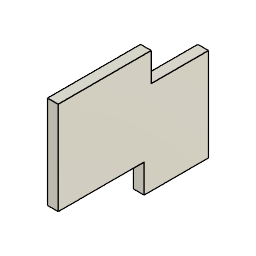
right_side_face_plate (Autodesk Fusion 360 design; units mm, degrees)
part number: 2025-10-03-12-31-24-970
Autodesk Fusion 360 part; units mm, degrees
sketch "Side Face Plate" plane through (0, 0, 0) normal (1, 0, 0) x (0, 1, 0)
  line L0 (0, 0) -> (168, 0)
  line L1 (168, 0) -> (168, 136)
  line L2 (168, 136) -> (0, 136)
  line L3 (0, 136) -> (0, 0)
  line L4 (168, 136) -> (104, 136)
  line L5 (104, 136) -> (104, 104)
  line L6 (104, 104) -> (168, 104)
  line L7 (168, 104) -> (168, 136)
  line L8 (0, 0) -> (96, 0)
  line L9 (96, 0) -> (96, 32)
  line L10 (96, 32) -> (0, 32)
  line L11 (0, 32) -> (0, 0)
  dimension "d4" = 136
  dimension "d5" = 168
  dimension "d14" = 32
  dimension "d15" = 64
  dimension "d18" = 32
  dimension "d19" = 96
  constraint horizontal L0
  constraint vertical L1
  constraint horizontal L2
  constraint vertical L3
  constraint coincident L0.start L3.end
  constraint horizontal L4
  constraint vertical L5
  constraint horizontal L6
  constraint vertical L7
  constraint horizontal L8
  constraint vertical L9
  constraint horizontal L10
  constraint vertical L11
  measures "d4" distance of L0.start L2.end
  measures "d5" distance of L0.start L0.end
  measures "d14" distance of L4 L6
  measures "d15" distance of L5 L7
  measures "d18" distance of L8 L10
  measures "d19" distance of L9 L11
extrude "Extrude1" add sketch "Side Face Plate" along normal blind 12 contours L0 L1 L2 L3 L5 L6 L9 L10
equation "block_size = 16 mm" comment "The size of the blocks used for the dimensions of the Minecraft Pig."
equation "pine_thickness = 12 mm" comment "The thickness of the pine boards used for the Minecraft Pig's body."
equation "side_face_plate_height = 10 * block_size - 2 * pine_thickness" comment "The height of the Side Face Plates that make up the Minecraft Pig's face."
equation "d4 = side_face_plate_height"
equation "d5 = side_face_plate_length"
equation "d6 = pine_thickness"
equation "side_face_plate_length = ( 8 * block_size - 2 * pine_thickness ) + 4 * block_size" comment "The length of the Side Face Plates that make up the Minecraft Pig's face."
equation "top_cutaway_height = 2 * block_size" comment "The height of the top cutaway in the Side Face Plates."
equation "top_cutaway_length = 4 * block_size" comment "The length of the top cutaway in the Side Face Plates."
equation "d14 = top_cutaway_height"
equation "d15 = top_cutaway_length"
equation "bottom_cutaway_height = 2 * block_size" comment "The height of the bottom cutaway in the Side Face Plates."
equation "bottom_cutaway_length = 6 * block_size" comment "The length of the bottom cutaway in the Side Face Plates."
equation "d18 = bottom_cutaway_height"
equation "d19 = bottom_cutaway_length"
named bodies: "Right Side Face Plate"
